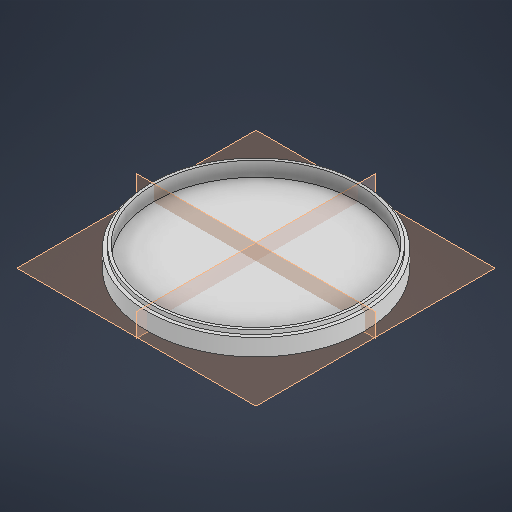
# Autodesk Inventor part: plate
Saved by Autodesk Inventor 2026 (Build 300175050, 175E)
## iProperties
Created: 2025-07-28
Part Number: plate
Material: Generic
Document SubType Name: Modeling
Designer: bruno
Density: 1 g/cm^3
Appearance: Default
Author: bruno
Autodesk Inventor part; units mm, degrees
sketch "Sketch1" plane through (0, 0, 0) normal (0, 1, 0) x (-1, 0, 0)
  circle A0 centre (0, 0) radius 51.5
  dimension "d0" = 103
  constraints: 1 centre point, 1 coincident
  measures "d0" diameter of A0
extrude "Extrusion1" add sketch "Sketch1" along normal blind 10
shell "Shell1" thickness 3 removed faces 1 at (13.8689, 10, -1.7627)
sketch "Sketch2" plane through (0, 10, 0) normal (0, 1, 0) x (1, 0, 0)
  circle A0 centre (0, 0) radius 51.5 projected
  circle A1 centre (0, 0) radius 48.5 projected
  circle A2 centre (0, 0) radius 51.5 projected
  circle A3 centre (0, 0) radius 49.8
  dimension "d4" = 1.3
  constraints: 1 centre point
  measures "d4" radial gap between concentric circles of A1 A3
extrude "Extrusion2" cut sketch "Sketch2" against normal blind 2 contours A0
body "Solid1"
